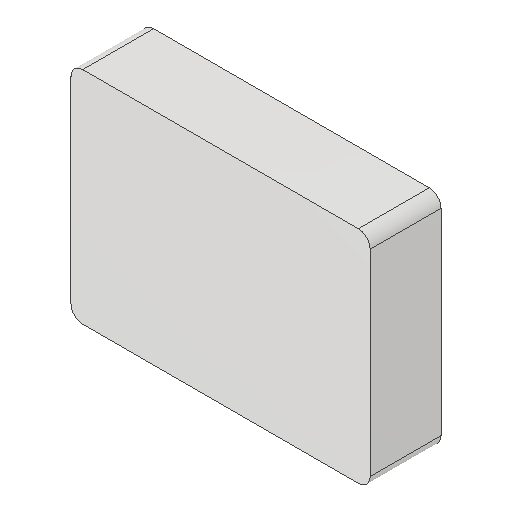
# Autodesk Inventor part: 3DP_PLA_Tray_for_unknown_parts
Saved by Autodesk Inventor 2026.1 (Build 301233000, 233)
## iProperties
Created: 2018-08-02
Part Number: 3DP_PLA_Tray_for_unknown_parts
Material: ABS Plastic
Document SubType Name: Modeling
Designer: Andrzej
Density: 1.06 g/cm^3
Appearance: Smooth - White
Author: Andrzej
Autodesk Inventor part; units mm, degrees
ref_plane "YZ Plane" through (0, 0, 0) normal (1, 0, 0) x (0, 1, 0)
ref_plane "XZ Plane" through (0, 0, 0) normal (0, 1, 0) x (-1, 0, 0)
ref_plane "XY Plane" through (0, 0, 0) normal (0, 0, 1) x (1, 0, 0)
sketch "Sketch1" plane through (0, 0, 0) normal (0, 0, 1) x (1, 0, 0)
  line L0 (-18.2588, 5.5059) -> (51.7412, 5.5059)
  line L1 (51.7412, 5.5059) -> (51.7412, -44.4941)
  line L2 (51.7412, -44.4941) -> (-18.2588, -44.4941)
  line L3 (-18.2588, -44.4941) -> (-18.2588, 5.5059)
  line L4 (54.7412, 8.5059) -> (-21.2588, 8.5059)
  line L5 (-21.2588, 8.5059) -> (-21.2588, -47.4941)
  line L6 (-21.2588, -47.4941) -> (54.7412, -47.4941)
  line L7 (54.7412, -47.4941) -> (54.7412, 8.5059)
  point P0 (0, 0)
  dimension "d0" = 70
  dimension "d1" = 50
  dimension "d2" = 3
  constraints: 16 end point, 4 parallel, 2 perpendicular, 1 horizontal, 3 other
  measures "d0" distance of L1.end L2.end
  measures "d1" distance of L0.end L1.end
  measures "d2" distance between parallel lines of L0 L4
extrude "Extrusion1" add sketch "Sketch1" along normal blind 3 contours L0 L1 L2 L3 | L7 L6 L5 L4
extrude "Extrusion2" add sketch "Sketch1" against normal blind 15
fillet "Fillet1" radius 3 8 edges at (51.7412, -44.4941, -7.5) (54.7412, -47.4941, -6) (54.7412, 8.5059, -6) (51.7412, 5.5059, -7.5) (-21.2588, 8.5059, -6) (-18.2588, 5.5059, -7.5) (-18.2588, -44.4941, -7.5) (-21.2588, -47.4941, -6)
body "Solid1"
